Autodesk Fusion 360 part; units mm, degrees
note: some values were not read from the file. Chosen so that the rebuilt part matches the saved one: where a step ends; which bodies a step acts on; which face or edge a step refers to. Set by a fixed rule: which sketch regions a step uses.
(part 2 of 5)
  spline S2 degree 5 poles (-10.814323, -5.434869) (-10.81447, -5.434944) (-10.814783, -5.435107) (-10.815312, -5.435384) (-10.816135, -5.43582) (-10.817359, -5.436478) (-10.818777, -5.437246) (-10.820385, -5.438125) (-10.822176, -5.439114) (-10.824145, -5.440212) (-10.826285, -5.441418) (-10.828592, -5.442732) (-10.831063, -5.444152) (-10.833693, -5.445679) (-10.836479, -5.447312) (-10.839418, -5.449051) (-10.842505, -5.450894) (-10.845736, -5.452842) (-10.849109, -5.454893) (-10.852619, -5.457048) (-10.856264, -5.459305) (-10.860042, -5.461665) (-10.863948, -5.464127) (-10.867979, -5.466691) (-10.872134, -5.469356) (-10.87641, -5.472121) (-10.880803, -5.474987) (-10.885311, -5.477953) (-10.889933, -5.481019) (-10.894664, -5.484184) (-10.899504, -5.487447) (-10.904449, -5.49081) (-10.909498, -5.49427) (-10.914649, -5.497828) (-10.919899, -5.501484) (-10.925246, -5.505237) (-10.930688, -5.509087) (-10.936224, -5.513033) (-10.941851, -5.517076) (-10.947568, -5.521214) (-10.953372, -5.525448) (-10.959263, -5.529778) (-10.965238, -5.534203) (-10.971295, -5.538722) (-10.977434, -5.543336) (-10.983652, -5.548044) (-10.989948, -5.552846) (-10.99632, -5.557742) (-11.002767, -5.562731) (-11.009287, -5.567813) (-11.015879, -5.572988) (-11.022541, -5.578256) (-11.029272, -5.583616) (-11.036071, -5.589068) (-11.042937, -5.594612) (-11.049867, -5.600248) (-11.056861, -5.605975) (-11.063918, -5.611793) (-11.071035, -5.617702) (-11.078213, -5.623702) (-11.085449, -5.629792) (-11.092744, -5.635973) (-11.100094, -5.642243) (-11.1075, -5.648603) (-11.11496, -5.655052) (-11.122474, -5.661591) (-11.130039, -5.668219) (-11.137655, -5.674935) (-11.145321, -5.68174) (-11.153036, -5.688634) (-11.160799, -5.695616) (-11.168609, -5.702685) (-11.176465, -5.709842) (-11.184366, -5.717087) (-11.192311, -5.724419) (-11.200299, -5.731838) (-11.208329, -5.739344) (-11.2164, -5.746937) (-11.224511, -5.754616) (-11.232662, -5.762381) (-11.240852, -5.770233) (-11.249079, -5.77817) (-11.257344, -5.786193) (-11.265644, -5.794301) (-11.273979, -5.802494) (-11.282349, -5.810773) (-11.290753, -5.819136) (-11.299189, -5.827584) (-11.307657, -5.836116) (-11.316157, -5.844732) (-11.324687, -5.853432) (-11.333247, -5.862217) (-11.341836, -5.871084) (-11.350453, -5.880036) (-11.359098, -5.88907) (-11.36777, -5.898187) (-11.376467, -5.907388) (-11.385191, -5.916671) (-11.393939, -5.926036) (-11.402711, -5.935483) (-11.411506, -5.945013) (-11.420324, -5.954624) (-11.429165, -5.964318) (-11.438026, -5.974092) (-11.446909, -5.983948) (-11.455812, -5.993885) (-11.464734, -6.003903) (-11.473675, -6.014002) (-11.482634, -6.024181) (-11.491612, -6.03444) (-11.500606, -6.04478) (-11.509617, -6.0552) (-11.518643, -6.065699) (-11.527685, -6.076278) (-11.536742, -6.086936) (-11.545813, -6.097674) (-11.554897, -6.108491) (-11.563995, -6.119386) (-11.573105, -6.13036) (-11.582227, -6.141413) (-11.59136, -6.152544) (-11.600505, -6.163753) (-11.60966, -6.17504) (-11.618824, -6.186405) (-11.627998, -6.197847) (-11.637181, -6.209367) (-11.646372, -6.220964) (-11.65557, -6.232638) (-11.664776, -6.244389) (-11.673989, -6.256217) (-11.683208, -6.26812) (-11.692433, -6.280101) (-11.701664, -6.292157) (-11.710899, -6.30429) (-11.720138, -6.316498) (-11.729382, -6.328781) (-11.738628, -6.34114) (-11.747878, -6.353575) (-11.757131, -6.366084) (-11.766385, -6.378668) (-11.775641, -6.391327) (-11.784898, -6.404061) (-11.794156, -6.416868) (-11.803415, -6.42975) (-11.812673, -6.442706) (-11.82193, -6.455736) (-11.831187, -6.468839) (-11.840442, -6.482016) (-11.849696, -6.495266) (-11.858947, -6.508589) (-11.868195, -6.521985) (-11.877441, -6.535453) (-11.886683, -6.548995) (-11.895921, -6.562608) (-11.905155, -6.576294) (-11.914384, -6.590052) (-11.923609, -6.603882) (-11.932827, -6.617783) (-11.94204, -6.631756) (-11.951247, -6.6458) (-11.960447, -6.659916) (-11.96964, -6.674102) (-11.978826, -6.688359) (-11.988004, -6.702687) (-11.997175, -6.717085) (-12.006336, -6.731553) (-12.015489, -6.746092) (-12.024633, -6.7607) (-12.033767, -6.775379) (-12.042891, -6.790127) (-12.052006, -6.804944) (-12.061109, -6.81983) (-12.070202, -6.834786) (-12.079283, -6.84981) (-12.088353, -6.864903) (-12.097411, -6.880065) (-12.106457, -6.895295) (-12.11549, -6.910593) (-12.12451, -6.925959) (-12.133517, -6.941393) (-12.14251, -6.956895) (-12.151489, -6.972464) (-12.160454, -6.9881) (-12.169405, -7.003804) (-12.17834, -7.019575) (-12.187261, -7.035412) (-12.196166, -7.051316) (-12.205055, -7.067287) (-12.213928, -7.083323) (-12.222785, -7.099426) (-12.231625, -7.115595) (-12.240448, -7.13183) (-12.249253, -7.14813) (-12.258041, -7.164495) (-12.266811, -7.180926) (-12.275563, -7.197422) (-12.284296, -7.213983) (-12.293011, -7.230609) (-12.301706, -7.247299) (-12.310382, -7.264053) (-12.319039, -7.280872) (-12.327675, -7.297755) (-12.336292, -7.314701) (-12.344887, -7.331712) (-12.353462, -7.348786) (-12.362016, -7.365923) (-12.370549, -7.383123) (-12.37906, -7.400387) (-12.387549, -7.417713) (-12.396017, -7.435102) (-12.404461, -7.452554) (-12.412883, -7.470068) (-12.421283, -7.487644) (-12.429659, -7.505282) (-12.438011, -7.522982) (-12.44634, -7.540743) (-12.454645, -7.558566) (-12.462926, -7.57645) (-12.471182, -7.594396) (-12.479414, -7.612402) (-12.48762, -7.63047) (-12.495802, -7.648598) (-12.503958, -7.666786) (-12.512088, -7.685035) (-12.520192, -7.703343) (-12.52827, -7.721712) (-12.536322, -7.74014) (-12.544347, -7.758628) (-12.552346, -7.777176) (-12.560317, -7.795783) (-12.568261, -7.814449) (-12.576177, -7.833174) (-12.584066, -7.851958) (-12.591926, -7.8708) (-12.599758, -7.889701) (-12.607562, -7.90866) (-12.615336, -7.927676) (-12.623082, -7.946751) (-12.630798, -7.965883) (-12.638485, -7.985073) (-12.646142, -8.004321) (-12.652245, -8.019765) (-12.656809, -8.031374) (-12.659845, -8.039125) (-12.661362, -8.043004) knots 0 0 0 0 0 0 0.00416667 0.00833333 0.0125 0.01666667 0.02083333 0.025 0.02916667 0.03333333 0.0375 0.04166667 0.04583333 0.05 0.05416667 0.05833333 0.0625 0.06666667 0.07083333 0.075 0.07916667 0.08333333 0.0875 0.09166667 0.09583333 0.1 0.10416667 0.10833333 0.1125 0.11666667 0.12083333 0.125 0.12916667 0.13333333 0.1375 0.14166667 0.14583333 0.15 0.15416667 0.15833333 0.1625 0.16666667 0.17083333 0.175 0.17916667 0.18333333 0.1875 0.19166667 0.19583333 0.2 0.20416667 0.20833333 0.2125 0.21666667 0.22083333 0.225 0.22916667 0.23333333 0.2375 0.24166667 0.24583333 0.25 0.25416667 0.25833333 0.2625 0.26666667 0.27083333 0.275 0.27916667 0.28333333 0.2875 0.29166667 0.29583333 0.3 0.30416667 0.30833333 0.3125 0.31666667 0.32083333 0.325 0.32916667 0.33333333 0.3375 0.34166667 0.34583333 0.35 0.35416667 0.35833333 0.3625 0.36666667 0.37083333 0.375 0.37916667 0.38333333 0.3875 0.39166667 0.39583333 0.4 0.40416667 0.40833333 0.4125 0.41666667 0.42083333 0.425 0.42916667 0.43333333 0.4375 0.44166667 0.44583333 0.45 0.45416667 0.45833333 0.4625 0.46666667 0.47083333 0.475 0.47916667 0.48333333 0.4875 0.49166667 0.49583333 0.5 0.50416667 0.50833333 0.5125 0.51666667 0.52083333 0.525 0.52916667 0.53333333 0.5375 0.54166667 0.54583333 0.55 0.55416667 0.55833333 0.5625 0.56666667 0.57083333 0.575 0.57916667 0.58333333 0.5875 0.59166667 0.59583333 0.6 0.60416667 0.60833333 0.6125 0.61666667 0.62083333 0.625 0.62916667 0.63333333 0.6375 0.64166667 0.64583333 0.65 0.65416667 0.65833333 0.6625 0.66666667 0.67083333 0.675 0.67916667 0.68333333 0.6875 0.69166667 0.69583333 0.7 0.70416667 0.70833333 0.7125 0.71666667 0.72083333 0.725 0.72916667 0.73333333 0.7375 0.74166667 0.74583333 0.75 0.75416667 0.75833333 0.7625 0.76666667 0.77083333 0.775 0.77916667 0.78333333 0.7875 0.79166667 0.79583333 0.8 0.80416667 0.80833333 0.8125 0.81666667 0.82083333 0.825 0.82916667 0.83333333 0.8375 0.84166667 0.84583333 0.85 0.85416667 0.85833333 0.8625 0.86666667 0.87083333 0.875 0.87916667 0.88333333 0.8875 0.89166667 0.89583333 0.9 0.90416667 0.90833333 0.9125 0.91666667 0.92083333 0.925 0.92916667 0.93333333 0.9375 0.94166667 0.94583333 0.95 0.95416667 0.95833333 0.9625 0.96666667 0.97083333 0.975 0.97916667 0.98333333 0.9875 0.99166667 0.99583333 1 1 1 1 1 1
  arc A3 (-12.661362, -8.043004) -> (-11.561927, -9.556246) centre (0, 0) ccw
  spline S3 degree 5 poles (-11.561927, -9.556246) (-11.55777, -9.556002) (-11.54946, -9.555509) (-11.537009, -9.554756) (-11.520435, -9.553725) (-11.499763, -9.55239) (-11.479137, -9.551009) (-11.458556, -9.549583) (-11.438022, -9.548111) (-11.417533, -9.546594) (-11.397091, -9.545031) (-11.376695, -9.543423) (-11.356346, -9.541769) (-11.336044, -9.540072) (-11.315789, -9.538329) (-11.295582, -9.536542) (-11.275422, -9.534711) (-11.255311, -9.532835) (-11.235248, -9.530916) (-11.215233, -9.528953) (-11.195267, -9.526947) (-11.17535, -9.524897) (-11.155482, -9.522803) (-11.135664, -9.520667) (-11.115895, -9.518488) (-11.096176, -9.516266) (-11.076507, -9.514002) (-11.056888, -9.511695) (-11.037321, -9.509346) (-11.017803, -9.506955) (-10.998338, -9.504522) (-10.978923, -9.502048) (-10.95956, -9.499533) (-10.940249, -9.496976) (-10.920989, -9.494378) (-10.901782, -9.491739) (-10.882628, -9.48906) (-10.863526, -9.486341) (-10.844478, -9.483581) (-10.825482, -9.480781) (-10.80654, -9.477941) (-10.787652, -9.475062) (-10.768818, -9.472144) (-10.750038, -9.469186) (-10.731313, -9.466189) (-10.712643, -9.463154) (-10.694027, -9.46008) (-10.675467, -9.456967) (-10.656962, -9.453817) (-10.638513, -9.450628) (-10.62012, -9.447403) (-10.601783, -9.444139) (-10.583503, -9.440839) (-10.565279, -9.437501) (-10.547113, -9.434127) (-10.529004, -9.430716) (-10.510952, -9.427269) (-10.492958, -9.423786) (-10.475023, -9.420267) (-10.457145, -9.416712) (-10.439326, -9.413122) (-10.421566, -9.409497) (-10.403865, -9.405837) (-10.386224, -9.402143) (-10.368642, -9.398414) (-10.35112, -9.394652) (-10.333658, -9.390855) (-10.316257, -9.387025) (-10.298916, -9.383161) (-10.281636, -9.379265) (-10.264417, -9.375335) (-10.24726, -9.371373) (-10.230165, -9.367379) (-10.213132, -9.363353) (-10.196161, -9.359295) (-10.179252, -9.355206) (-10.162407, -9.351085) (-10.145624, -9.346934) (-10.128905, -9.342752) (-10.11225, -9.33854) (-10.095658, -9.334298) (-10.079131, -9.330026) (-10.062668, -9.325724) (-10.04627, -9.321394) (-10.029938, -9.317034) (-10.01367, -9.312646) (-9.997468, -9.30823) (-9.981332, -9.303786) (-9.965262, -9.299314) (-9.949259, -9.294815) (-9.933323, -9.290289) (-9.917453, -9.285736) (-9.901651, -9.281157) (-9.885917, -9.276551) (-9.87025, -9.271921) (-9.854652, -9.267264) (-9.839122, -9.262583) (-9.823661, -9.257877) (-9.808269, -9.253146) (-9.792947, -9.248392) (-9.777694, -9.243614) (-9.762512, -9.238812) (-9.747399, -9.233988) (-9.732357, -9.229141) (-9.717387, -9.224271) (-9.702487, -9.21938) (-9.687659, -9.214467) (-9.672903, -9.209534) (-9.658219, -9.204579) (-9.643607, -9.199604) (-9.629068, -9.194609) (-9.614602, -9.189594) (-9.60021, -9.18456) (-9.585891, -9.179507) (-9.571647, -9.174436) (-9.557477, -9.169346) (-9.543381, -9.164239) (-9.52936, -9.159115) (-9.515415, -9.153974) (-9.501546, -9.148817) (-9.487752, -9.143643) (-9.474035, -9.138454) (-9.460394, -9.13325) (-9.446831, -9.128031) (-9.433345, -9.122798) (-9.419936, -9.117551) (-9.406605, -9.112291) (-9.393353, -9.107018) (-9.380179, -9.101733) (-9.367085, -9.096436) (-9.35407, -9.091127) (-9.341134, -9.085807) (-9.328279, -9.080477) (-9.315504, -9.075136) (-9.30281, -9.069786) (-9.290197, -9.064428) (-9.277666, -9.05906) (-9.265216, -9.053685) (-9.252849, -9.048302) (-9.240564, -9.042912) (-9.228362, -9.037516) (-9.216244, -9.032114) (-9.204209, -9.026706) (-9.192259, -9.021294) (-9.180393, -9.015877) (-9.168612, -9.010457) (-9.156916, -9.005034) (-9.145305, -8.999608) (-9.133781, -8.99418) (-9.122344, -8.988751) (-9.110993, -8.983322) (-9.099729, -8.977892) (-9.088553, -8.972462) (-9.077465, -8.967034) (-9.066466, -8.961607) (-9.055555, -8.956183) (-9.044734, -8.950762) (-9.034003, -8.945345) (-9.023361, -8.939932) (-9.012811, -8.934524) (-9.002351, -8.929122) (-8.991983, -8.923727) (-8.981707, -8.918338) (-8.971523, -8.912958) (-8.961432, -8.907586) (-8.951434, -8.902223) (-8.94153, -8.896871) (-8.93172, -8.891529) (-8.922005, -8.886199) (-8.912385, -8.880881) (-8.90286, -8.875577) (-8.893432, -8.870287) (-8.8841, -8.865012) (-8.874866, -8.859752) (-8.865729, -8.854509) (-8.85669, -8.849283) (-8.84775, -8.844076) (-8.838909, -8.838888) (-8.830167, -8.83372) (-8.821526, -8.828573) (-8.812986, -8.823448) (-8.804547, -8.818346) (-8.79621, -8.813268) (-8.787975, -8.808215) (-8.779843, -8.803187) (-8.771815, -8.798187) (-8.763891, -8.793215) (-8.756071, -8.788271) (-8.748357, -8.783358) (-8.740749, -8.778476) (-8.733248, -8.773627) (-8.725853, -8.76881) (-8.718567, -8.764029) (-8.711389, -8.759284) (-8.70432, -8.754575) (-8.697362, -8.749905) (-8.690513, -8.745275) (-8.683776, -8.740685) (-8.677151, -8.736138) (-8.670638, -8.731634) (-8.664239, -8.727175) (-8.657954, -8.722763) (-8.651784, -8.718398) (-8.64573, -8.714083) (-8.639792, -8.709819) (-8.633971, -8.705607) (-8.628269, -8.701448) (-8.622685, -8.697346) (-8.617221, -8.693301) (-8.611878, -8.689314) (-8.606656, -8.685389) (-8.601557, -8.681526) (-8.596582, -8.677727) (-8.59173, -8.673994) (-8.587004, -8.67033) (-8.582405, -8.666735) (-8.577933, -8.663213) (-8.573589, -8.659766) (-8.569376, -8.656394) (-8.565292, -8.653102) (-8.561341, -8.64989) (-8.557523, -8.646762) (-8.553838, -8.64372) (-8.55029, -8.640766) (-8.546878, -8.637903) (-8.543605, -8.635134) (-8.540471, -8.632461) (-8.537477, -8.629887) (-8.534627, -8.627416) (-8.53192, -8.62505) (-8.529358, -8.622792) (-8.526944, -8.620647) (-8.524679, -8.618617) (-8.522565, -8.616707) (-8.520602, -8.614918) (-8.518794, -8.613255) (-8.517141, -8.611722) (-8.515647, -8.610324) (-8.514314, -8.609067) (-8.513145, -8.607956) (-8.512142, -8.606994) (-8.511472, -8.606347) (-8.511045, -8.60593) (-8.510794, -8.605682) (-8.510677, -8.605566) knots -1 -1 -1 -1 -1 -1 -0.99583333 -0.99166667 -0.9875 -0.98333333 -0.97916667 -0.975 -0.97083333 -0.96666667 -0.9625 -0.95833333 -0.95416667 -0.95 -0.94583333 -0.94166667 -0.9375 -0.93333333 -0.92916667 -0.925 -0.92083333 -0.91666667 -0.9125 -0.90833333 -0.90416667 -0.9 -0.89583333 -0.89166667 -0.8875 -0.88333333 -0.87916667 -0.875 -0.87083333 -0.86666667 -0.8625 -0.85833333 -0.85416667 -0.85 -0.84583333 -0.84166667 -0.8375 -0.83333333 -0.82916667 -0.825 -0.82083333 -0.81666667 -0.8125 -0.80833333 -0.80416667 -0.8 -0.79583333 -0.79166667 -0.7875 -0.78333333 -0.77916667 -0.775 -0.77083333 -0.76666667 -0.7625 -0.75833333 -0.75416667 -0.75 -0.74583333 -0.74166667 -0.7375 -0.73333333 -0.72916667 -0.725 -0.72083333 -0.71666667 -0.7125 -0.70833333 -0.70416667 -0.7 -0.69583333 -0.69166667 -0.6875 -0.68333333 -0.67916667 -0.675 -0.67083333 -0.66666667 -0.6625 -0.65833333 -0.65416667 -0.65 -0.64583333 -0.64166667 -0.6375 -0.63333333 -0.62916667 -0.625 -0.62083333 -0.61666667 -0.6125 -0.60833333 -0.60416667 -0.6 -0.59583333 -0.59166667 -0.5875 -0.58333333 -0.57916667 -0.575 -0.57083333 -0.56666667 -0.5625 -0.55833333 -0.55416667 -0.55 -0.54583333 -0.54166667 -0.5375 -0.53333333 -0.52916667 -0.525 -0.52083333 -0.51666667 -0.5125 -0.50833333 -0.50416667 -0.5 -0.49583333 -0.49166667 -0.4875 -0.48333333 -0.47916667 -0.475 -0.47083333 -0.46666667 -0.4625 -0.45833333 -0.45416667 -0.45 -0.44583333 -0.44166667 -0.4375 -0.43333333 -0.42916667 -0.425 -0.42083333 -0.41666667 -0.4125 -0.40833333 -0.40416667 -0.4 -0.39583333 -0.39166667 -0.3875 -0.38333333 -0.37916667 -0.375 -0.37083333 -0.36666667 -0.3625 -0.35833333 -0.35416667 -0.35 -0.34583333 -0.34166667 -0.3375 -0.33333333 -0.32916667 -0.325 -0.32083333 -0.31666667 -0.3125 -0.30833333 -0.30416667 -0.3 -0.29583333 -0.29166667 -0.2875 -0.28333333 -0.27916667 -0.275 -0.27083333 -0.26666667 -0.2625 -0.25833333 -0.25416667 -0.25 -0.24583333 -0.24166667 -0.2375 -0.23333333 -0.22916667 -0.225 -0.22083333 -0.21666667 -0.2125 -0.20833333 -0.20416667 -0.2 -0.19583333 -0.19166667 -0.1875 -0.18333333 -0.17916667 -0.175 -0.17083333 -0.16666667 -0.1625 -0.15833333 -0.15416667 -0.15 -0.14583333 -0.14166667 -0.1375 -0.13333333 -0.12916667 -0.125 -0.12083333 -0.11666667 -0.1125 -0.10833333 -0.10416667 -0.1 -0.09583333 -0.09166667 -0.0875 -0.08333333 -0.07916667 -0.075 -0.07083333 -0.06666667 -0.0625 -0.05833333 -0.05416667 -0.05 -0.04583333 -0.04166667 -0.0375 -0.03333333 -0.02916667 -0.025 -0.02083333 -0.01666667 -0.0125 -0.00833333 -0.00416667 0 0 0 0 0 0
  line L6 (-8.510677, -8.605566) -> (-8.509717, -8.604614)
  line L7 (-8.509717, -8.604614) -> (-6.592267, -6.665781)
  arc A4 (-6.592267, -6.665781) -> (-4.302412, -8.329458) centre (0, 0) ccw
  line L8 (-4.302412, -8.329458) -> (-5.553827, -10.752194)
  line L9 (-5.553827, -10.752194) -> (-5.554435, -10.753401)
  spline S4 degree 5 poles (-5.554435, -10.753401) (-5.55451, -10.753548) (-5.554668, -10.753864) (-5.554933, -10.754399) (-5.555342, -10.755235) (-5.555946, -10.756487) (-5.556641, -10.757942) (-5.557425, -10.759598) (-5.558293, -10.761451) (-5.559241, -10.763497) (-5.560263, -10.76573) (-5.561358, -10.768149) (-5.562521, -10.770751) (-5.563752, -10.773532) (-5.565046, -10.776491) (-5.566402, -10.779625) (-5.567815, -10.78293) (-5.569285, -10.786405) (-5.570808, -10.790047) (-5.572381, -10.793854) (-5.574003, -10.797823) (-5.575672, -10.801952) (-5.577385, -10.80624) (-5.57914, -10.810684) (-5.580935, -10.815282) (-5.582768, -10.820033) (-5.584638, -10.824933) (-5.586542, -10.829983) (-5.588479, -10.835179) (-5.590446, -10.840521) (-5.592443, -10.846006) (-5.594468, -10.851633) (-5.596519, -10.8574) (-5.598594, -10.863306) (-5.600692, -10.869349) (-5.602812, -10.875528) (-5.604952, -10.881842) (-5.607111, -10.888288) (-5.609288, -10.894866) (-5.61148, -10.901575) (-5.613687, -10.908412) (-5.615908, -10.915377) (-5.618141, -10.922469) (-5.620385, -10.929686) (-5.62264, -10.937027) (-5.624903, -10.94449) (-5.627174, -10.952076) (-5.629451, -10.959782) (-5.631734, -10.967608) (-5.634022, -10.975552) (-5.636313, -10.983613) (-5.638606, -10.991791) (-5.640902, -11.000084) (-5.643197, -11.008491) (-5.645493, -11.017012) (-5.647787, -11.025645) (-5.650079, -11.034389) (-5.652368, -11.043244) (-5.654653, -11.052208) (-5.656933, -11.061281) (-5.659208, -11.070461) (-5.661477, -11.079749) (-5.663738, -11.089142) (-5.665991, -11.09864) (-5.668235, -11.108243) (-5.67047, -11.117949) (-5.672695, -11.127758) (-5.674909, -11.137668) (-5.677111, -11.14768) (-5.679301, -11.157792) (-5.681478, -11.168003) (-5.683641, -11.178313) (-5.685789, -11.188721) (-5.687923, -11.199226) (-5.69004, -11.209828) (-5.692142, -11.220525) (-5.694226, -11.231317) (-5.696293, -11.242204) (-5.698342, -11.253184) (-5.700372, -11.264258) (-5.702383, -11.275423) (-5.704373, -11.286681) (-5.706344, -11.298029) (-5.708293, -11.309467) (-5.71022, -11.320995) (-5.712126, -11.332612) (-5.714009, -11.344318) (-5.715868, -11.356111) (-5.717704, -11.367991) (-5.719516, -11.379958) (-5.721303, -11.39201) (-5.723065, -11.404148) (-5.724801, -11.416371) (-5.726511, -11.428678) (-5.728195, -11.441068) (-5.729851, -11.453541) (-5.73148, -11.466097) (-5.733081, -11.478734) (-5.734654, -11.491453) (-5.736197, -11.504252) (-5.737711, -11.517132) (-5.739196, -11.530091) (-5.740651, -11.543129) (-5.742074, -11.556245) (-5.743467, -11.56944) (-5.744829, -11.582712) (-5.746159, -11.596061) (-5.747457, -11.609487) (-5.748722, -11.622988) (-5.749954, -11.636565) (-5.751153, -11.650216) (-5.752318, -11.663942) (-5.75345, -11.677742) (-5.754547, -11.691615) (-5.755609, -11.705562) (-5.756636, -11.71958) (-5.757628, -11.733671) (-5.758583, -11.747833) (-5.759503, -11.762066) (-5.760386, -11.77637) (-5.761233, -11.790743) (-5.762042, -11.805187) (-5.762814, -11.819699) (-5.763549, -11.83428) (-5.764245, -11.84893) (-5.764902, -11.863647) (-5.765522, -11.878431) (-5.766102, -11.893283) (-5.766643, -11.9082) (-5.767144, -11.923184) (-5.767605, -11.938234) (-5.768027, -11.953348) (-5.768407, -11.968527) (-5.768748, -11.983771) (-5.769047, -11.999078) (-5.769305, -12.014449) (-5.769521, -12.029883) (-5.769696, -12.045379) (-5.769828, -12.060938) (-5.769918, -12.076559) (-5.769966, -12.09224) (-5.769971, -12.107983) (-5.769932, -12.123787) (-5.769851, -12.13965) (-5.769725, -12.155574) (-5.769556, -12.171556) (-5.769343, -12.187598) (-5.769086, -12.203698) (-5.768784, -12.219857) (-5.768437, -12.236073) (-5.768045, -12.252347) (-5.767608, -12.268677) (-5.767126, -12.285065) (-5.766598, -12.301509) (-5.766024, -12.318008) (-5.765404, -12.334563) (-5.764738, -12.351174) (-5.764025, -12.367839) (-5.763265, -12.384558) (-5.762459, -12.401332) (-5.761605, -12.418159) (-5.760704, -12.43504) (-5.759755, -12.451974) (-5.758759, -12.46896) (-5.757715, -12.485998) (-5.756622, -12.503089) (-5.755482, -12.52023) (-5.754292, -12.537423) (-5.753054, -12.554667) (-5.751768, -12.571962) (-5.750432, -12.589306) (-5.749047, -12.606701) (-5.747612, -12.624144) (-5.746128, -12.641637) (-5.744594, -12.659179) (-5.74301, -12.676769) (-5.741377, -12.694407) (-5.739692, -12.712093) (-5.737958, -12.729827) (-5.736173, -12.747607) (-5.734337, -12.765434) (-5.73245, -12.783308) (-5.730512, -12.801228) (-5.728523, -12.819193) (-5.726482, -12.837204) (-5.72439, -12.85526) (-5.722246, -12.873361) (-5.72005, -12.891506) (-5.717802, -12.909696) (-5.715503, -12.927929) (-5.71315, -12.946206) (-5.710746, -12.964526) (-5.708289, -12.982889) (-5.705779, -13.001294) (-5.703216, -13.019742) (-5.700601, -13.038232) (-5.697932, -13.056763) (-5.69521, -13.075336) (-5.692434, -13.093949) (-5.689605, -13.112604) (-5.686723, -13.131299) (-5.683786, -13.150033) (-5.680796, -13.168808) (-5.677752, -13.187622) (-5.674653, -13.206476) (-5.6715, -13.225368) (-5.668293, -13.244299) (-5.665032, -13.263268) (-5.661716, -13.282275) (-5.658345, -13.30132) (-5.654919, -13.320402) (-5.651438, -13.339522) (-5.647902, -13.358678) (-5.644311, -13.37787) (-5.640665, -13.397099) (-5.636963, -13.416364) (-5.633206, -13.435665) (-5.629393, -13.455001) (-5.625524, -13.474372) (-5.6216, -13.493778) (-5.61762, -13.513219) (-5.613583, -13.532693) (-5.609491, -13.552202) (-5.605342, -13.571744) (-5.601137, -13.59132) (-5.596875, -13.610929) (-5.592557, -13.63057) (-5.588183, -13.650245) (-5.583752, -13.669951) (-5.579264, -13.68969) (-5.574719, -13.709461) (-5.570117, -13.729263) (-5.565458, -13.749096) (-5.560742, -13.76896) (-5.555969, -13.788854) (-5.551138, -13.808779) (-5.54625, -13.828734) (-5.541305, -13.848718) (-5.536301, -13.868732) (-5.531241, -13.888775) (-5.526122, -13.908848) (-5.521981, -13.924929) (-5.51885, -13.937004) (-5.516751, -13.945059) (-5.515698, -13.949089) knots 0 0 0 0 0 0 0.00416667 0.00833333 0.0125 0.01666667 0.02083333 0.025 0.02916667 0.03333333 0.0375 0.04166667 0.04583333 0.05 0.05416667 0.05833333 0.0625 0.06666667 0.07083333 0.075 0.07916667 0.08333333 0.0875 0.09166667 0.09583333 0.1 0.10416667 0.10833333 0.1125 0.11666667 0.12083333 0.125 0.12916667 0.13333333 0.1375 0.14166667 0.14583333 0.15 0.15416667 0.15833333 0.1625 0.16666667 0.17083333 0.175 0.17916667 0.18333333 0.1875 0.19166667 0.19583333 0.2 0.20416667 0.20833333 0.2125 0.21666667 0.22083333 0.225 0.22916667 0.23333333 0.2375 0.24166667 0.24583333 0.25 0.25416667 0.25833333 0.2625 0.26666667 0.27083333 0.275 0.27916667 0.28333333 0.2875 0.29166667 0.29583333 0.3 0.30416667 0.30833333 0.3125 0.31666667 0.32083333 0.325 0.32916667 0.33333333 0.3375 0.34166667 0.34583333 0.35 0.35416667 0.35833333 0.3625 0.36666667 0.37083333 0.375 0.37916667 0.38333333 0.3875 0.39166667 0.39583333 0.4 0.40416667 0.40833333 0.4125 0.41666667 0.42083333 0.425 0.42916667 0.43333333 0.4375 0.44166667 0.44583333 0.45 0.45416667 0.45833333 0.4625 0.46666667 0.47083333 0.475 0.47916667 0.48333333 0.4875 0.49166667 0.49583333 0.5 0.50416667 0.50833333 0.5125 0.51666667 0.52083333 0.525 0.52916667 0.53333333 0.5375 0.54166667 0.54583333 0.55 0.55416667 0.55833333 0.5625 0.56666667 0.57083333 0.575 0.57916667 0.58333333 0.5875 0.59166667 0.59583333 0.6 0.60416667 0.60833333 0.6125 0.61666667 0.62083333 0.625 0.62916667 0.63333333 0.6375 0.64166667 0.64583333 0.65 0.65416667 0.65833333 0.6625 0.66666667 0.67083333 0.675 0.67916667 0.68333333 0.6875 0.69166667 0.69583333 0.7 0.70416667 0.70833333 0.7125 0.71666667 0.72083333 0.725 0.72916667 0.73333333 0.7375 0.74166667 0.74583333 0.75 0.75416667 0.75833333 0.7625 0.76666667 0.77083333 0.775 0.77916667 0.78333333 0.7875 0.79166667 0.79583333 0.8 0.80416667 0.80833333 0.8125 0.81666667 0.82083333 0.825 0.82916667 0.83333333 0.8375 0.84166667 0.84583333 0.85 0.85416667 0.85833333 0.8625 0.86666667 0.87083333 0.875 0.87916667 0.88333333 0.8875 0.89166667 0.89583333 0.9 0.90416667 0.90833333 0.9125 0.91666667 0.92083333 0.925 0.92916667 0.93333333 0.9375 0.94166667 0.94583333 0.95 0.95416667 0.95833333 0.9625 0.96666667 0.97083333 0.975 0.97916667 0.98333333 0.9875 0.99166667 0.99583333 1 1 1 1 1 1
  arc A5 (-5.515698, -13.949089) -> (-3.736775, -14.527096) centre (0, 0) ccw
  spline S5 degree 5 poles (-3.736775, -14.527096) (-3.733555, -14.524455) (-3.727122, -14.519172) (-3.717491, -14.511244) (-3.704689, -14.500667) (-3.68875, -14.487437) (-3.672874, -14.474196) (-3.657063, -14.460945) (-3.641315, -14.447684) (-3.625631, -14.434414) (-3.610012, -14.421134) (-3.594457, -14.407845) (-3.578965, -14.394546) (-3.563539, -14.381239) (-3.548176, -14.367924) (-3.532879, -14.354601) (-3.517646, -14.34127) (-3.502478, -14.327931) (-3.487374, -14.314586) (-3.472336, -14.301233) (-3.457363, -14.287874) (-3.442454, -14.274509) (-3.427611, -14.261138) (-3.412833, -14.24776) (-3.398121, -14.234377) (-3.383474, -14.220989) (-3.368893, -14.207596) (-3.354377, -14.194199) (-3.339927, -14.180797) (-3.325542, -14.167391) (-3.311224, -14.153981) (-3.296971, -14.140567) (-3.282785, -14.127151) (-3.268665, -14.113732) (-3.254611, -14.10031) (-3.240623, -14.086885) (-3.226701, -14.073459) (-3.212846, -14.060031) (-3.199058, -14.046602) (-3.185336, -14.033172) (-3.171681, -14.019741) (-3.158092, -14.006309) (-3.144571, -13.992878) (-3.131116, -13.979446) (-3.117728, -13.966015) (-3.104408, -13.952585) (-3.091154, -13.939156) (-3.077968, -13.925729) (-3.064849, -13.912304) (-3.051798, -13.89888) (-3.038814, -13.885459) (-3.025897, -13.872041) (-3.013048, -13.858626) (-3.000267, -13.845214) (-2.987553, -13.831806) (-2.974907, -13.818403) (-2.962329, -13.805003) (-2.94982, -13.791609) (-2.937378, -13.77822) (-2.925004, -13.764836) (-2.912698, -13.751458) (-2.900461, -13.738086) (-2.888291, -13.724721) (-2.876191, -13.711363) (-2.864158, -13.698012) (-2.852194, -13.684668) (-2.840299, -13.671333) (-2.828472, -13.658006) (-2.816714, -13.644688) (-2.805025, -13.631379) (-2.793404, -13.618079) (-2.781853, -13.604789) (-2.77037, -13.591509) (-2.758956, -13.57824) (-2.747612, -13.564982) (-2.736336, -13.551735) (-2.72513, -13.5385) (-2.713992, -13.525277) (-2.702924, -13.512066) (-2.691926, -13.498869) (-2.680997, -13.485684) (-2.670137, -13.472514) (-2.659347, -13.459357) (-2.648626, -13.446215) (-2.637975, -13.433088) (-2.627393, -13.419977) (-2.616881, -13.40688) (-2.606439, -13.393801) (-2.596067, -13.380737) (-2.585765, -13.367691) (-2.575532, -13.354662) (-2.56537, -13.341651) (-2.555277, -13.328658) (-2.545254, -13.315684) (-2.535302, -13.302729) (-2.52542, -13.289793) (-2.515607, -13.276878) (-2.505865, -13.263983) (-2.496194, -13.251109) (-2.486592, -13.238256) (-2.477061, -13.225425) (-2.4676, -13.212616) (-2.45821, -13.199831) (-2.44889, -13.187068) (-2.43964, -13.174329) (-2.430461, -13.161614) (-2.421353, -13.148924) (-2.412315, -13.136259) (-2.403347, -13.123619) (-2.39445, -13.111006) (-2.385624, -13.098419) (-2.376869, -13.085859) (-2.368184, -13.073327) (-2.35957, -13.060823) (-2.351027, -13.048347) (-2.342554, -13.035901) (-2.334153, -13.023484) (-2.325822, -13.011097) (-2.317562, -12.998741) (-2.309373, -12.986417) (-2.301254, -12.974123) (-2.293207, -12.961863) (-2.28523, -12.949635) (-2.277325, -12.93744) (-2.26949, -12.92528) (-2.261726, -12.913153) (-2.254033, -12.901062) (-2.246411, -12.889007) (-2.23886, -12.876988) (-2.23138, -12.865005) (-2.223971, -12.85306) (-2.216633, -12.841153) (-2.209366, -12.829285) (-2.20217, -12.817455) (-2.195045, -12.805666) (-2.18799, -12.793917) (-2.181007, -12.782209) (-2.174095, -12.770542) (-2.167253, -12.758918) (-2.160483, -12.747337) (-2.153783, -12.735799) (-2.147155, -12.724306) (-2.140597, -12.712857) (-2.13411, -12.701454) (-2.127694, -12.690097) (-2.121349, -12.678788) (-2.115074, -12.667525) (-2.108871, -12.656312) (-2.102738, -12.645147) (-2.096676, -12.634032) (-2.090684, -12.622967) (-2.084763, -12.611954) (-2.078913, -12.600992) (-2.073133, -12.590083) (-2.067424, -12.579228) (-2.061786, -12.568426) (-2.056218, -12.55768) (-2.05072, -12.54699) (-2.045293, -12.536356) (-2.039935, -12.525779) (-2.034649, -12.515261) (-2.029432, -12.504801) (-2.024286, -12.494402) (-2.019209, -12.484063) (-2.014203, -12.473786) (-2.009267, -12.463571) (-2.0044, -12.453419) (-1.999604, -12.443331) (-1.994877, -12.433309) (-1.99022, -12.423352) (-1.985632, -12.413463) (-1.981114, -12.403641) (-1.976665, -12.393888) (-1.972286, -12.384205) (-1.967976, -12.374593) (-1.963735, -12.365053) (-1.959562, -12.355585) (-1.955459, -12.346191) (-1.951425, -12.336872) (-1.94746, -12.327629) (-1.943563, -12.318463) (-1.939734, -12.309375) (-1.935974, -12.300366) (-1.932282, -12.291437) (-1.928658, -12.28259) (-1.925102, -12.273826) (-1.921614, -12.265146) (-1.918194, -12.25655) (-1.914841, -12.248041) (-1.911556, -12.23962) (-1.908337, -12.231287) (-1.905186, -12.223045) (-1.902102, -12.214894) (-1.899084, -12.206835) (-1.896133, -12.198871) (-1.893248, -12.191003) (-1.89043, -12.183231) (-1.887677, -12.175558) (-1.88499, -12.167985) (-1.882368, -12.160514) (-1.879812, -12.153145) (-1.877321, -12.145881) (-1.874895, -12.138724) (-1.872533, -12.131674) (-1.870236, -12.124733) (-1.868002, -12.117905) (-1.865833, -12.111189) (-1.863727, -12.104588) (-1.861684, -12.098103) (-1.859705, -12.091738) (-1.857788, -12.085493) (-1.855933, -12.07937) (-1.854141, -12.073372) (-1.85241, -12.067501) (-1.850741, -12.061759) (-1.849132, -12.056147) (-1.847584, -12.050669) (-1.846097, -12.045327) (-1.844669, -12.040123) (-1.843301, -12.035059) (-1.841992, -12.030138) (-1.840742, -12.025363) (-1.83955, -12.020736) (-1.838415, -12.016261) (-1.837338, -12.011939) (-1.836317, -12.007775) (-1.835353, -12.00377) (-1.834444, -11.999929) (-1.83359, -11.996254) (-1.832791, -11.992748) (-1.832046, -11.989416) (-1.831354, -11.986262) (-1.830714, -11.983288) (-1.830127, -11.9805) (-1.82959, -11.9779) (-1.829104, -11.975491) (-1.828669, -11.97328) (-1.828282, -11.97127) (-1.827942, -11.96947) (-1.82765, -11.967884) (-1.827403, -11.966516) (-1.827242, -11.965599) (-1.827142, -11.96501) (-1.827084, -11.964662) (-1.827058, -11.964499) knots -1 -1 -1 -1 -1 -1 -0.99583333 -0.99166667 -0.9875 -0.98333333 -0.97916667 -0.975 -0.97083333 -0.96666667 -0.9625 -0.95833333 -0.95416667 -0.95 -0.94583333 -0.94166667 -0.9375 -0.93333333 -0.92916667 -0.925 -0.92083333 -0.91666667 -0.9125 -0.90833333 -0.90416667 -0.9 -0.89583333 -0.89166667 -0.8875 -0.88333333 -0.87916667 -0.875 -0.87083333 -0.86666667 -0.8625 -0.85833333 -0.85416667 -0.85 -0.84583333 -0.84166667 -0.8375 -0.83333333 -0.82916667 -0.825 -0.82083333 -0.81666667 -0.8125 -0.80833333 -0.80416667 -0.8 -0.79583333 -0.79166667 -0.7875 -0.78333333 -0.77916667 -0.775 -0.77083333 -0.76666667 -0.7625 -0.75833333 -0.75416667 -0.75 -0.74583333 -0.74166667 -0.7375 -0.73333333 -0.72916667 -0.725 -0.72083333 -0.71666667 -0.7125 -0.70833333 -0.70416667 -0.7 -0.69583333 -0.69166667 -0.6875 -0.68333333 -0.67916667 -0.675 -0.67083333 -0.66666667 -0.6625 -0.65833333 -0.65416667 -0.65 -0.64583333 -0.64166667 -0.6375 -0.63333333 -0.62916667 -0.625 -0.62083333 -0.61666667 -0.6125 -0.60833333 -0.60416667 -0.6 -0.59583333 -0.59166667 -0.5875 -0.58333333 -0.57916667 -0.575 -0.57083333 -0.56666667 -0.5625 -0.55833333 -0.55416667 -0.55 -0.54583333 -0.54166667 -0.5375 -0.53333333 -0.52916667 -0.525 -0.52083333 -0.51666667 -0.5125 -0.50833333 -0.50416667 -0.5 -0.49583333 -0.49166667 -0.4875 -0.48333333 -0.47916667 -0.475 -0.47083333 -0.46666667 -0.4625 -0.45833333 -0.45416667 -0.45 -0.44583333 -0.44166667 -0.4375 -0.43333333 -0.42916667 -0.425 -0.42083333 -0.41666667 -0.4125 -0.40833333 -0.40416667 -0.4 -0.39583333 -0.39166667 -0.3875 -0.38333333 -0.37916667 -0.375 -0.37083333 -0.36666667 -0.3625 -0.35833333 -0.35416667 -0.35 -0.34583333 -0.34166667 -0.3375 -0.33333333 -0.32916667 -0.325 -0.32083333 -0.31666667 -0.3125 -0.30833333 -0.30416667 -0.3 -0.29583333 -0.29166667 -0.2875 -0.28333333 -0.27916667 -0.275 -0.27083333 -0.26666667 -0.2625 -0.25833333 -0.25416667 -0.25 -0.24583333 -0.24166667 -0.2375 -0.23333333 -0.22916667 -0.225 -0.22083333 -0.21666667 -0.2125 -0.20833333 -0.20416667 -0.2 -0.19583333 -0.19166667 -0.1875 -0.18333333 -0.17916667 -0.175 -0.17083333 -0.16666667 -0.1625 -0.15833333 -0.15416667 -0.15 -0.14583333 -0.14166667 -0.1375 -0.13333333 -0.12916667 -0.125 -0.12083333 -0.11666667 -0.1125 -0.10833333 -0.10416667 -0.1 -0.09583333 -0.09166667 -0.0875 -0.08333333 -0.07916667 -0.075 -0.07083333 -0.06666667 -0.0625 -0.05833333 -0.05416667 -0.05 -0.04583333 -0.04166667 -0.0375 -0.03333333 -0.02916667 -0.025 -0.02083333 -0.01666667 -0.0125 -0.00833333 -0.00416667 0 0 0 0 0 0
  line L10 (-1.827058, -11.964499) -> (-1.82684, -11.963165)
  line L11 (-1.82684, -11.963165) -> (-1.415208, -9.267568)
  arc A6 (-1.415208, -9.267568) -> (1.415208, -9.267568) centre (0, 0) ccw
  line L12 (1.415208, -9.267568) -> (1.82684, -11.963165)
  line L13 (1.82684, -11.963165) -> (1.827058, -11.964499)
  spline S6 degree 5 poles (1.827058, -11.964499) (1.827084, -11.964662) (1.827142, -11.96501) (1.827242, -11.965599) (1.827403, -11.966516) (1.82765, -11.967884) (1.827942, -11.96947) (1.828282, -11.97127) (1.828669, -11.97328) (1.829104, -11.975491) (1.82959, -11.9779) (1.830127, -11.9805) (1.830714, -11.983288) (1.831354, -11.986262) (1.832046, -11.989416) (1.832791, -11.992748) (1.83359, -11.996254) (1.834444, -11.999929) (1.835353, -12.00377) (1.836317, -12.007775) (1.837338, -12.011939) (1.838415, -12.016261) (1.83955, -12.020736) (1.840742, -12.025363) (1.841992, -12.030138) (1.843301, -12.035059) (1.844669, -12.040123) (1.846097, -12.045327) (1.847584, -12.050669) (1.849132, -12.056147) (1.850741, -12.061759) (1.85241, -12.067501) (1.854141, -12.073372) (1.855933, -12.07937) (1.857788, -12.085493) (1.859705, -12.091738) (1.861684, -12.098103) (1.863727, -12.104588) (1.865833, -12.111189) (1.868002, -12.117905) (1.870236, -12.124733) (1.872533, -12.131674) (1.874895, -12.138724) (1.877321, -12.145881) (1.879812, -12.153145) (1.882368, -12.160514) (1.88499, -12.167985) (1.887677, -12.175558) (1.89043, -12.183231) (1.893248, -12.191003) (1.896133, -12.198871) (1.899084, -12.206835) (1.902102, -12.214894) (1.905186, -12.223045) (1.908337, -12.231287) (1.911556, -12.23962) (1.914841, -12.248041) (1.918194, -12.25655) (1.921614, -12.265146) (1.925102, -12.273826) (1.928658, -12.28259) (1.932282, -12.291437) (1.935974, -12.300366) (1.939734, -12.309375) (1.943563, -12.318463) (1.94746, -12.327629) (1.951425, -12.336872) (1.955459, -12.346191) (1.959562, -12.355585) (1.963735, -12.365053) (1.967976, -12.374593) (1.972286, -12.384205) (1.976665, -12.393888) (1.981114, -12.403641) (1.985632, -12.413463) (1.99022, -12.423352) (1.994877, -12.433309) (1.999604, -12.443331) (2.0044, -12.453419) (2.009267, -12.463571) (2.014203, -12.473786) (2.019209, -12.484063) (2.024286, -12.494402) (2.029432, -12.504801) (2.034649, -12.515261) (2.039935, -12.525779) (2.045293, -12.536356) (2.05072, -12.54699) (2.056218, -12.55768) (2.061786, -12.568426) (2.067424, -12.579228) (2.073133, -12.590083) (2.078913, -12.600992) (2.084763, -12.611954) (2.090684, -12.622967) (2.096676, -12.634032) (2.102738, -12.645147) (2.108871, -12.656312) (2.115074, -12.667525) (2.121349, -12.678788) (2.127694, -12.690097) (2.13411, -12.701454) (2.140597, -12.712857) (2.147155, -12.724306) (2.153783, -12.735799) (2.160483, -12.747337) (2.167253, -12.758918) (2.174095, -12.770542) (2.181007, -12.782209) (2.18799, -12.793917) (2.195045, -12.805666) (2.20217, -12.817455) (2.209366, -12.829285) (2.216633, -12.841153) (2.223971, -12.85306) (2.23138, -12.865005) (2.23886, -12.876988) (2.246411, -12.889007) (2.254033, -12.901062) (2.261726, -12.913153) (2.26949, -12.92528) (2.277325, -12.93744) (2.28523, -12.949635) (2.293207, -12.961863) (2.301254, -12.974123) (2.309373, -12.986417) (2.317562, -12.998741) (2.325822, -13.011097) (2.334153, -13.023484) (2.342554, -13.035901) (2.351027, -13.048347) (2.35957, -13.060823) (2.368184, -13.073327) (2.376869, -13.085859) (2.385624, -13.098419) (2.39445, -13.111006) (2.403347, -13.123619) (2.412315, -13.136259) (2.421353, -13.148924) (2.430461, -13.161614) (2.43964, -13.174329) (2.44889, -13.187068) (2.45821, -13.199831) (2.4676, -13.212616) (2.477061, -13.225425) (2.486592, -13.238256) (2.496194, -13.251109) (2.505865, -13.263983) (2.515607, -13.276878) (2.52542, -13.289793) (2.535302, -13.302729) (2.545254, -13.315684) (2.555277, -13.328658) (2.56537, -13.341651) (2.575532, -13.354662) (2.585765, -13.367691) (2.596067, -13.380737) (2.606439, -13.393801) (2.616881, -13.40688) (2.627393, -13.419977) (2.637975, -13.433088) (2.648626, -13.446215) (2.659347, -13.459357) (2.670137, -13.472514) (2.680997, -13.485684) (2.691926, -13.498869) (2.702924, -13.512066) (2.713992, -13.525277) (2.72513, -13.5385) (2.736336, -13.551735) (2.747612, -13.564982) (2.758956, -13.57824) (2.77037, -13.591509) (2.781853, -13.604789) (2.793404, -13.618079) (2.805025, -13.631379) (2.816714, -13.644688) (2.828472, -13.658006) (2.840299, -13.671333) (2.852194, -13.684668) (2.864158, -13.698012) (2.876191, -13.711363) (2.888291, -13.724721) (2.900461, -13.738086) (2.912698, -13.751458) (2.925004, -13.764836) (2.937378, -13.77822) (2.94982, -13.791609) (2.962329, -13.805003) (2.974907, -13.818403) (2.987553, -13.831806) (3.000267, -13.845214) (3.013048, -13.858626) (3.025897, -13.872041) (3.038814, -13.885459) (3.051798, -13.89888) (3.064849, -13.912304) (3.077968, -13.925729) (3.091154, -13.939156) (3.104408, -13.952585) (3.117728, -13.966015) (3.131116, -13.979446) (3.144571, -13.992878) (3.158092, -14.006309) (3.171681, -14.019741) (3.185336, -14.033172) (3.199058, -14.046602) (3.212846, -14.060031) (3.226701, -14.073459) (3.240623, -14.086885) (3.254611, -14.10031) (3.268665, -14.113732) (3.282785, -14.127151) (3.296971, -14.140567) (3.311224, -14.153981) (3.325542, -14.167391) (3.339927, -14.180797) (3.354377, -14.194199) (3.368893, -14.207596) (3.383474, -14.220989) (3.398121, -14.234377) (3.412833, -14.24776) (3.427611, -14.261138) (3.442454, -14.274509) (3.457363, -14.287874) (3.472336, -14.301233) (3.487374, -14.314586) (3.502478, -14.327931) (3.517646, -14.34127) (3.532879, -14.354601) (3.548176, -14.367924) (3.563539, -14.381239) (3.578965, -14.394546) (3.594457, -14.407845) (3.610012, -14.421134) (3.625631, -14.434414) (3.641315, -14.447684) (3.657063, -14.460945) (3.672874, -14.474196) (3.68875, -14.487437) (3.704689, -14.500667) (3.717491, -14.511244) (3.727122, -14.519172) (3.733555, -14.524455) (3.736775, -14.527096) knots 0 0 0 0 0 0 0.00416667 0.00833333 0.0125 0.01666667 0.02083333 0.025 0.02916667 0.03333333 0.0375 0.04166667 0.04583333 0.05 0.05416667 0.05833333 0.0625 0.06666667 0.07083333 0.075 0.07916667 0.08333333 0.0875 0.09166667 0.09583333 0.1 0.10416667 0.10833333 0.1125 0.11666667 0.12083333 0.125 0.12916667 0.13333333 0.1375 0.14166667 0.14583333 0.15 0.15416667 0.15833333 0.1625 0.16666667 0.17083333 0.175 0.17916667 0.18333333 0.1875 0.19166667 0.19583333 0.2 0.20416667 0.20833333 0.2125 0.21666667 0.22083333 0.225 0.22916667 0.23333333 0.2375 0.24166667 0.24583333 0.25 0.25416667 0.25833333 0.2625 0.26666667 0.27083333 0.275 0.27916667 0.28333333 0.2875 0.29166667 0.29583333 0.3 0.30416667 0.30833333 0.3125 0.31666667 0.32083333 0.325 0.32916667 0.33333333 0.3375 0.34166667 0.34583333 0.35 0.35416667 0.35833333 0.3625 0.36666667 0.37083333 0.375 0.37916667 0.38333333 0.3875 0.39166667 0.39583333 0.4 0.40416667 0.40833333 0.4125 0.41666667 0.42083333 0.425 0.42916667 0.43333333 0.4375 0.44166667 0.44583333 0.45 0.45416667 0.45833333 0.4625 0.46666667 0.47083333 0.475 0.47916667 0.48333333 0.4875 0.49166667 0.49583333 0.5 0.50416667 0.50833333 0.5125 0.51666667 0.52083333 0.525 0.52916667 0.53333333 0.5375 0.54166667 0.54583333 0.55 0.55416667 0.55833333 0.5625 0.56666667 0.57083333 0.575 0.57916667 0.58333333 0.5875 0.59166667 0.59583333 0.6 0.60416667 0.60833333 0.6125 0.61666667 0.62083333 0.625 0.62916667 0.63333333 0.6375 0.64166667 0.64583333 0.65 0.65416667 0.65833333 0.6625 0.66666667 0.67083333 0.675 0.67916667 0.68333333 0.6875 0.69166667 0.69583333 0.7 0.70416667 0.70833333 0.7125 0.71666667 0.72083333 0.725 0.72916667 0.73333333 0.7375 0.74166667 0.74583333 0.75 0.75416667 0.75833333 0.7625 0.76666667 0.77083333 0.775 0.77916667 0.78333333 0.7875 0.79166667 0.79583333 0.8 0.80416667 0.80833333 0.8125 0.81666667 0.82083333 0.825 0.82916667 0.83333333 0.8375 0.84166667 0.84583333 0.85 0.85416667 0.85833333 0.8625 0.86666667 0.87083333 0.875 0.87916667 0.88333333 0.8875 0.89166667 0.89583333 0.9 0.90416667 0.90833333 0.9125 0.91666667 0.92083333 0.925 0.92916667 0.93333333 0.9375 0.94166667 0.94583333 0.95 0.95416667 0.95833333 0.9625 0.96666667 0.97083333 0.975 0.97916667 0.98333333 0.9875 0.99166667 0.99583333 1 1 1 1 1 1
  arc A7 (3.736775, -14.527096) -> (5.515698, -13.949089) centre (0, 0) ccw